PLATE_LV_SIDE_CON (Autodesk Fusion 360 design; units mm, degrees)
Autodesk Fusion 360 part; units mm, degrees
note: some values were not read from the file. Set by a fixed rule: which sketch regions a step uses.
sketch "Esquisse1" plane through (0, 0, 0) normal (0, 0, 1) x (1, 0, 0)
  line L0 (103, -50) -> (-103, -50)
  line L1 (-103, -50) -> (-103, 50)
  line L2 (-103, 50) -> (103, 50)
  line L3 (103, 50) -> (103, -50)
  line L4 (103, -50) -> (-103, 50) construction
  line L5 (-103, -50) -> (103, 50) construction
  line L6 (-100, -53) -> (100, -53)
  line L7 (100, -53) -> (100, 53)
  line L8 (100, 53) -> (-100, 53)
  line L9 (-100, 53) -> (-100, -53)
  line L10 (-100, -53) -> (100, 53) construction
  line L11 (100, -53) -> (-100, 53) construction
  dimension "d1" = 206
  dimension "d2" = 100
  dimension "d41" = 200
  dimension "d42" = 106
  constraint horizontal L0
  constraint perpendicular L0 L1
  constraint parallel L0 L2
  constraint parallel L1 L3
  constraint coincident L4 origin
  constraint coincident L5 origin
  constraint horizontal L6
  constraint perpendicular L6 L7
  constraint parallel L6 L8
  constraint parallel L7 L9
  constraint coincident L10 origin
  constraint coincident L11 origin
  measures "d1" distance of L1.end L2.end
  measures "d2" distance of L0.end L1.end
  measures "d41" distance of L7.end L8.end
  measures "d42" distance of L6.end L7.end
extrude "Extrusion1" add sketch "Esquisse1" along normal blind 3
sketch "Esquisse3" plane through (0, 0, 3) normal (0, 0, 1) x (-1, 0, 0)
  line L0 (100, -50) -> (103, -50)
  line L1 (103, -50) -> (103, 50)
  line L2 (103, 50) -> (100, 50)
  line L3 (-103, 50) -> (-103, -50)
  line L4 (-4.6, -3.6) -> (-92.4, -3.6)
  line L5 (-92.4, -3.6) -> (-92.4, 38.6)
  line L6 (-92.4, 38.6) -> (-4.6, 38.6)
  line L7 (-4.6, 38.6) -> (-4.6, -3.6)
  line L8 (-4.6, -3.6) -> (-92.4, 38.6) construction
  line L9 (-92.4, -3.6) -> (-4.6, 38.6) construction
  line L10 (-2, -10) -> (-95, -10)
  line L11 (-95, -10) -> (-95, 45)
  line L12 (-95, 45) -> (-2, 45)
  line L13 (-2, 45) -> (-2, -10)
  line L14 (-2, -10) -> (-95, 45) construction
  line L15 (-95, -10) -> (-2, 45) construction
  line L16 (103, 50) -> (103, -50)
  line L17 (-100, -50) -> (-100, -53)
  line L18 (-100, -53) -> (100, -53)
  line L19 (100, -53) -> (100, -50)
  line L20 (100, 50) -> (100, 53)
  line L21 (100, 53) -> (-100, 53)
  line L22 (-100, 53) -> (-100, 50)
  line L23 (-100, 50) -> (-103, 50)
  line L24 (-103, -50) -> (-100, -50)
  circle A0 centre (-2, 45) radius 1.5
  circle A1 centre (-95, 45) radius 1.5
  circle A2 centre (-95, -10) radius 1.5
  circle A3 centre (-2, -10) radius 1.5
  line L25 (15.5, 40.6667) -> (31.5, 40.6667)
  line L26 (35.5, 36.6667) -> (35.5, 12.6667)
  line L27 (31.5, 8.6667) -> (15.5, 8.6667)
  line L28 (11.5, 12.6667) -> (11.5, 36.6667)
  line L29 (11.5, 40.6667) -> (35.5, 8.6667) construction
  line L30 (35.5, 40.6667) -> (11.5, 8.6667) construction
  circle A4 centre (31.5, 28.6667) radius 2.5
  circle A5 centre (15.5, 28.6667) radius 2.5
  arc A6 (31.5, 8.6667) -> (35.5, 12.6667) centre (31.5, 12.6667) ccw
  arc A7 (11.5, 12.6667) -> (15.5, 8.6667) centre (15.5, 12.6667) ccw
  arc A8 (15.5, 40.6667) -> (11.5, 36.6667) centre (15.5, 36.6667) ccw
  arc A9 (35.5, 36.6667) -> (31.5, 40.6667) centre (31.5, 36.6667) ccw
  circle A10 centre (23.5, 16.6667) radius 5.125
  line L31 (100, 53) -> (-100, 53)
  line L32 (14, -6) -> (86, -6)
  line L33 (86, -6) -> (86, -44)
  line L34 (86, -44) -> (14, -44)
  line L35 (14, -44) -> (14, -6)
  line L36 (14, -6) -> (86, -44) construction
  line L37 (86, -6) -> (14, -44) construction
  line L38 (-92.4, 30.15) -> (-96.1, 30.15)
  line L39 (-96.1, 30.15) -> (-96.1, 4.85)
  line L40 (-96.1, 4.85) -> (-92.4, 4.85)
  line L41 (-92.4, 4.85) -> (-92.4, 30.15)
  line L42 (-92.4, 30.15) -> (-96.1, 4.85) construction
  line L43 (-96.1, 30.15) -> (-92.4, 4.85) construction
  line L44 (-92.4, 4.85) -> (-96.1, 7.8397)
  line L45 (-92.4, 30.15) -> (-96.1, 27.8397)
  line L46 (14, -19) -> (12, -19)
  line L47 (12, -19) -> (12, -31)
  line L48 (12, -31) -> (14, -31)
  line L49 (14, -31) -> (14, -19)
  line L50 (14, -19) -> (12, -31) construction
  line L51 (12, -19) -> (14, -31) construction
  line L52 (50, -25) -> (50, -44)
  line L53 (86, -19) -> (88, -19)
  line L54 (86, -31) -> (86, -19)
  line L55 (88, -31) -> (86, -31)
  line L56 (88, -19) -> (86, -31) construction
  line L57 (88, -19) -> (88, -31)
  line L58 (86, -19) -> (88, -31) construction
  point P0 (-48.5, 17.5)
  point P1 (-48.5, 17.5)
  point P2 (23.5, 24.6667)
  point P3 (50, -25)
  point P4 (-94.25, 17.5)
  point P5 (13, -25)
  point P6 (87, -25)
  dimension "d26" = 3
  dimension "d27" = 100
  dimension "d30" = 87.8
  dimension "d31" = 42.2
  dimension "d34" = 93
  dimension "d35" = 55
  dimension "d44" = 3
  dimension "d45" = 3
  dimension "d46" = 3
  dimension "d47" = 3
  dimension "d48" = 24
  dimension "d49" = 32
  dimension "d50" = 5
  dimension "d51" = 12
  dimension "d52" = 4
  dimension "d53" = 5
  dimension "d54" = 12
  dimension "d55" = 4
  dimension "d56" = 4
  dimension "d57" = 4
  dimension "d58" = 4
  dimension "d59" = 4
  dimension "d60" = 10.25
  dimension "d61" = 8
  dimension "d62" = 12
  dimension "d63" = 8
  dimension "d64" = 8
  dimension "d65" = 72
  dimension "d66" = 38
  dimension "d67" = 53
  dimension "d68" = 200
  dimension "d69" = 79.5
  dimension "d70" = 28
  dimension "d71" = 36.3333
  dimension "d72" = 25.3
  dimension "d73" = 3.7
  dimension "d74" = 21.1
  dimension "d75" = 20
  dimension "d76" = 12
  dimension "d77" = 2
  dimension "d78" = 19
  constraint horizontal L4
  constraint perpendicular L4 L5
  constraint parallel L4 L6
  constraint parallel L5 L7
  constraint coincident L8 P1
  constraint coincident L9 P1
  constraint horizontal L10
  constraint perpendicular L10 L11
  constraint parallel L10 L12
  constraint parallel L11 L13
  constraint coincident L14 P1
  constraint coincident L15 P1
  constraint coincident P1 P0
  constraint coincident L12.end L13.start
  constraint coincident L11.end L12.start
  constraint coincident L10.end L11.start
  constraint coincident L10.start L13.end
  constraint horizontal L25
  constraint perpendicular L25 L26
  constraint parallel L25 L27
  constraint parallel L26 L28
  constraint coincident L29 P2
  constraint coincident L30 P2
  constraint coincident L29.end L26
  constraint coincident L29.end L27
  constraint tangent L26 A6
  constraint tangent L27 A6
  constraint coincident L30.end L27
  constraint coincident L30.end L28
  constraint tangent L27 A7
  constraint tangent L28 A7
  constraint coincident L29.start L28
  constraint coincident L29.start L25
  constraint tangent L28 A8
  constraint tangent L25 A8
  constraint coincident L30.start L25
  constraint coincident L30.start L26
  constraint tangent L25 A9
  constraint tangent L26 A9
  constraint horizontal L32
  constraint perpendicular L32 L33
  constraint parallel L32 L34
  constraint parallel L33 L35
  constraint coincident L36 P3
  constraint coincident L37 P3
  constraint horizontal L38
  constraint perpendicular L38 L39
  constraint parallel L38 L40
  constraint parallel L39 L41
  constraint coincident L42 P4
  constraint coincident L43 P4
  constraint collinear L5 L41
  constraint coincident L39 L44.end
  constraint coincident L39 L45.end
  constraint horizontal L46
  constraint perpendicular L46 L47
  constraint parallel L46 L48
  constraint parallel L47 L49
  constraint coincident L50 P5
  constraint coincident L51 P5
  constraint collinear L35 L49
  constraint coincident P3 L52.start
  constraint midpoint L34 L52.end
  constraint symmetric L46.start L52 L53.start
  constraint symmetric L46.end L52 L53.end
  constraint symmetric L47.end L52 L55.start
  constraint symmetric L48.end L52 L54.start
  constraint symmetric P5 L52 P6
  measures "d26" distance of L0.start L0.end
  measures "d27" distance of L0.end L1.end
  measures "d30" distance of L5.end L6.end
  measures "d31" distance of L4.end L5.end
  measures "d34" distance of L11.end L12.end
  measures "d35" distance of L10.end L11.end
  measures "d44" diameter of A0
  measures "d45" diameter of A1
  measures "d46" diameter of A2
  measures "d47" diameter of A3
  measures "d48" distance of L29.end L30.end
  measures "d49" distance of L30.start L29.end
  measures "d50" diameter of A4
  measures "d51" distance of L25 A4.centre
  measures "d52" distance of L26 A4.centre
  measures "d53" diameter of A5
  measures "d54" distance of L25 A5.centre
  measures "d55" distance of L28 A5.centre
  measures "d56" radius of A6
  measures "d57" radius of A7
  measures "d58" radius of A8
  measures "d59" radius of A9
  measures "d60" diameter of A10
  measures "d61" distance of L27 A10.centre
  measures "d62" distance of L28 A10.centre
  measures "d63" distance of L11.end L31
  measures "d64" distance of L3 L11.end
  measures "d65" distance of L33.end L34.end
  measures "d66" distance of L32.end L33.end
  measures "d67" distance of L16 P3
  measures "d68" distance of L20.end L21.end
  measures "d69" distance of L16 A10.centre
  measures "d70" distance of L18 P3
  measures "d71" distance of L21 A10.centre
  measures "d72" distance of L38 L40
  measures "d73" distance of L39.end L40.end
  measures "d74" distance of L6 P4
  measures "d75" distance of L44.end L45.end
  measures "d76" distance of L46.end L47.end
  measures "d77" distance of L46.start L46.end
  measures "d78" distance of L32 P5
extrude "Extrusion3" cut sketch "Esquisse3" against normal blind 3 contours L4 L5 L6 L7 L41 | L5 L11 L41 L44 L45 | L11 L39 L44 L45 | L10 L11 A2 | L10 L11 A2 | L11 L12 A1 | L11 L12 A1 | L10 L13 A3 | L10 L13 A3 | L12 L13 A0 | L12 L13 A0 | A4 | A5 | A10 | L32 L33 L34 L35 L49 L54 | L35 L46 L47 L48 L49 | L33 L53 L54 L55 L57
equation "d30 = 87.3 mm + 0.5 mm"
equation "d31 = 41.7 mm + 0.5 mm"
equation "d52 = ( d48 - 16 mm ) / 2"
equation "d54 = d51"
equation "d55 = d52"
equation "d57 = d56"
equation "d58 = d57"
equation "d59 = d56"
equation "d62 = d48 / 2"
equation "d67 = d68 / 4 + 3 mm"
equation "d69 = d67 * 3 / 2"
equation "d70 = d27 / 4 + 3 mm"
equation "d71 = d27 / 3 + 3 mm"
equation "d74 = d31 / 2"
equation "d78 = d66 / 2"
